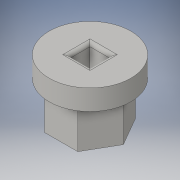
# Autodesk Inventor part: Flex Wheel Connector
Saved by Autodesk Inventor 2016 (Build 200138000, 138)
## iProperties
Created: 2019-06-07
Part Number: Flex Wheel Connector
Material: Generic
Document SubType Name: Modeling
Designer: Afnan
Density: 1 g/cm^3
Appearance: Default
Author: Afnan
Autodesk Inventor part; units mm, degrees
ref_plane "YZ Plane" through (0, 0, 0) normal (1, 0, 0) x (0, 1, 0)
ref_plane "XZ Plane" through (0, 0, 0) normal (0, 1, 0) x (-1, 0, 0)
ref_plane "XY Plane" through (0, 0, 0) normal (0, 0, 1) x (1, 0, 0)
sketch "Sketch1" plane through (0, 0, 0) normal (0, 1, 0) x (-1, 0, 0)
  line L0 (-5.4846, 0) -> (-2.7423, 4.7498)
  line L1 (-2.7423, 4.7498) -> (2.7423, 4.7498)
  line L2 (2.7423, 4.7498) -> (5.4846, 0)
  line L3 (5.4846, 0) -> (2.7423, -4.7498)
  line L4 (2.7423, -4.7498) -> (-2.7423, -4.7498)
  line L5 (-2.7423, -4.7498) -> (-5.4846, 0)
  line L6 (-2.5957, -4.4958) -> (2.5957, -4.4958)
  line L7 (2.5957, -4.4958) -> (5.1913, 0)
  line L8 (5.1913, 0) -> (2.5957, 4.4958)
  line L9 (2.5957, 4.4958) -> (-2.5957, 4.4958)
  line L10 (-2.5957, 4.4958) -> (-5.1913, 0)
  line L11 (-5.1913, 0) -> (-2.5957, -4.4958)
  point P0 (0, 0)
  point P1 (0, 0)
  dimension "d0" = 9.4996
  dimension "d1" = 0.254
  constraints: 24 end point, 1 coincident, 18 other
  measures "d0" distance between parallel lines of L1 L4
  measures "d1" distance between parallel lines of L4 L6
extrude "Extrusion1" add sketch "Sketch1" along normal blind 6.35 contours L11 L10 L9 L8 L7 L6
sketch "Sketch2" plane through (0, 6.35, 0) normal (0, 1, 0) x (1, 0, 0)
  circle A0 centre (0, 0) radius 6.35
  line L0 (1.6002, -1.6002) -> (-1.6002, -1.6002)
  line L1 (-1.6002, -1.6002) -> (-1.6002, 1.6002)
  line L2 (-1.6002, 1.6002) -> (1.6002, 1.6002)
  line L3 (1.6002, 1.6002) -> (1.6002, -1.6002)
  line L4 (1.6002, -1.6002) -> (-1.6002, 1.6002) construction
  line L5 (-1.6002, -1.6002) -> (1.6002, 1.6002) construction
  dimension "d4" = 12.7
  dimension "d5" = 3.2004
  dimension "d6" = 3.2004
  constraints: 12 end point, 2 midpoint, 2 parallel, 1 centre point, 1 coincident, 1 horizontal, 1 perpendicular
  measures "d4" diameter of A0
  measures "d5" distance of L1.end L2.end
  measures "d6" distance of L0.end L1.end
extrude "Extrusion2" add sketch "Sketch2" along normal blind 3.175
sketch "Sketch3" plane through (0, 9.525, 0) normal (0, 1, 0) x (1, 0, 0)
  line L0 (-1.6002, -1.6002) -> (-1.6002, 1.6002) projected
  line L1 (-1.6002, 1.6002) -> (-1.6002, -1.6002) projected
  line L2 (-1.6002, -1.6002) -> (1.6002, -1.6002) projected
  line L3 (1.6002, -1.6002) -> (1.6002, 1.6002) projected
  line L4 (1.6002, 1.6002) -> (-1.6002, 1.6002) projected
  point P0 (0, 0)
extrude "Extrusion3" cut sketch "Sketch3" against normal through all
fillet "Fillet1" radius 0.5292 4 edges at (0, 9.525, -1.6002) (1.6002, 9.525, 0) (-1.6002, 9.525, 0) (0, 9.525, 1.6002)
body "Solid1"
